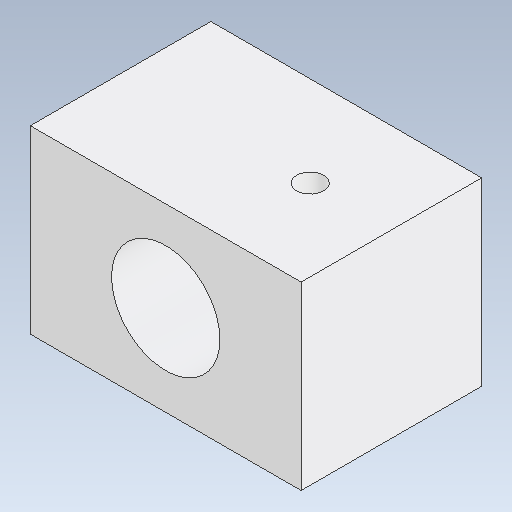
# Autodesk Inventor part: Bearing10
Saved by Autodesk Inventor 2020.5 (Build 245400000, 400)
## iProperties
Created: 2020-02-29
Part Number: Bearing10
Document SubType Name: Modeling
Designer: Administrator
Density: 7.85 g/cm^3
Material: Acero, carbono
Appearance: White
Mass: 75.4859 g
Surface Area: 38.5012 cm^2
Volume: 9.61604 cm^3
Author: Administrator
Autodesk Inventor part; units mm, degrees
ref_plane "YZ Plane" through (0, 0, 0) normal (1, 0, 0) x (0, 1, 0)
ref_plane "XZ Plane" through (0, 0, 0) normal (0, 1, 0) x (-1, 0, 0)
ref_plane "XY Plane" through (0, 0, 0) normal (0, 0, 1) x (1, 0, 0)
sketch "Sketch1" plane through (0, 0, 0) normal (0, 0, 1) x (1, 0, 0)
  circle A0 centre (0, 0) radius 6
  line L0 (10, 10) -> (10, -10)
  line L1 (10, -10) -> (-10, -10)
  line L2 (-10, -10) -> (-10, 10)
  line L3 (-10, 10) -> (10, 10)
  dimension "d0" = 12
  dimension "d1" = 20
  constraints: 8 end point, 1 centre point, 1 coincident, 10 other
  measures "d0" diameter of A0
  measures "d1" distance of L2.end L0.start
extrude "Extrusion1" add sketch "Sketch1" along normal blind 20
sketch "Sketch2" plane through (-10, -10, 0) normal (0, -1, 0) x (1, 0, 0)
  line L0 (7.9561, 12.9375) -> (13.8857, 12.9375) construction
  line L1 (13.8857, 12.9375) -> (13.8857, 9.2988) construction
  line L2 (13.8857, 9.2988) -> (7.9561, 9.2988) construction
  line L3 (7.9561, 9.2988) -> (7.9561, 12.9375) construction
  point P0 (10, 0)
  constraints: 2 other
sketch "Sketch3" plane through (-10, -10, 0) normal (0, -1, 0) x (1, 0, 0)
  line L0 (0, 0) -> (0, 20) projected
  line L1 (20, 0) -> (20, 20) projected
  line L2 (0, 20) -> (-5, 20)
  line L3 (-5, 20) -> (-5, 0)
  line L4 (-5, 0) -> (0, 0)
  line L5 (0, 0) -> (0, 20)
  line L6 (20, 0) -> (20, 20) projected
  line L7 (20, 20) -> (25, 20)
  line L8 (25, 20) -> (25, 0)
  line L9 (25, 0) -> (20, 0)
  line L10 (20, 0) -> (20, 20)
  point P0 (10, 0)
  dimension "d4" = 30
  constraints: 16 end point, 4 parallel, 3 equal length, 2 horizontal, 2 perpendicular
  measures "d4" distance between parallel lines of L8 L3
extrude "Extrusion2" add sketch "Sketch3" against normal up to surface (20 mm away)
sketch "Sketch4" plane through (-15, -10, 0) normal (0, -1, 0) x (1, 0, 0)
  line L0 (21, 0) -> (21, 20) projected
  line L1 (9, 0) -> (9, 20) projected
  circle A0 centre (21, 10) radius 1.5
  point P0 (15, 0)
  dimension "d7" = 3
  constraints: 1 centre point, 1 midpoint
  measures "d7" diameter of A0
extrude "Extrusion3" cut sketch "Sketch4" against normal through all
body "Solid1"
